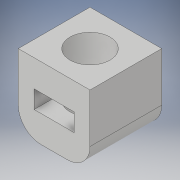
# Autodesk Inventor part: YMountB
Saved by Autodesk Inventor 2018 (Build 220112000, 112)
## iProperties
Created: 2020-03-14
Part Number: YMountB
Material: Generic
Document SubType Name: Modeling
Designer: natha
Density: 1 g/cm^3
Appearance: Default
Author: natha
Autodesk Inventor part; units mm, degrees
ref_plane "YZ Plane" through (0, 0, 0) normal (1, 0, 0) x (0, 1, 0)
ref_plane "XZ Plane" through (0, 0, 0) normal (0, 1, 0) x (-1, 0, 0)
ref_plane "XY Plane" through (0, 0, 0) normal (0, 0, 1) x (1, 0, 0)
sketch "Sketch1" plane through (0, 0, 0) normal (0, 1, 0) x (-1, 0, 0)
  line L0 (0, 0) -> (40, 0)
  line L1 (40, 0) -> (40, -40)
  line L2 (40, -40) -> (0, -40)
  line L3 (0, -40) -> (0, 0)
  circle A0 centre (20, -20) radius 11.15
  dimension "d0" = 40
  dimension "d1" = 40
  dimension "d2" = 22.3
  dimension "d3" = 20
  dimension "d4" = 20
  constraints: 8 end point, 2 parallel, 1 centre point, 1 horizontal, 1 perpendicular
  measures "d0" distance of L1.end L2.end
  measures "d1" distance of L0.end L1.end
  measures "d2" diameter of A0
  measures "d3" distance from line of L1 A0.centre
  measures "d4" distance from line of L2 A0.centre
extrude "Extrusion1" add sketch "Sketch1" along normal blind 40
fillet "Fillet1" radius 12.7 2 edges at (0, 0, -20) (-40, 0, -20)
sketch "Sketch2" plane through (-40, 40, 0) normal (0, 0, 1) x (1, 0, 0)
  line L0 (8.85, -15) -> (31.15, -15)
  line L1 (31.15, -15) -> (31.15, -25)
  line L2 (31.15, -25) -> (8.85, -25)
  line L3 (8.85, -25) -> (8.85, -15)
  line L4 (8.85, -15) -> (31.15, -25) construction
  line L5 (31.15, -15) -> (8.85, -25) construction
  line L6 (40, -27.3) -> (40, 0) projected
  line L7 (27.3, -40) -> (12.7, -40) projected
  point P0 (40, -40)
  point P1 (20, -20)
  dimension "d8" = 20
  dimension "d9" = 22.3
  dimension "d10" = 10
  dimension "d11" = 15
  constraints: 12 end point, 2 midpoint, 2 parallel, 1 horizontal, 1 perpendicular
  measures "d8" distance from line of L6 point (20, -20)
  measures "d9" distance between parallel lines of L3 L1
  measures "d10" distance between parallel lines of L0 L2
  measures "d11" distance between parallel lines of L7 L2
extrude "Extrusion2" cut sketch "Sketch2" against normal blind 20
body "Solid1"
